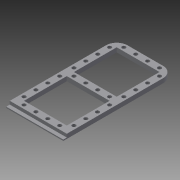
# Autodesk Inventor part: large edition 3 open
Saved by Autodesk Inventor 2015 (Build 190159000, 159)
## iProperties
Created: 2015-06-08
Part Number: large edition 3 open
Material: Generic
Document SubType Name: Modeling
Designer: Jason
Density: 1 g/cm^3
Appearance: Default
Author: Jason
Autodesk Inventor part; units mm, degrees
ref_plane "YZ Plane" through (0, 0, 0) normal (1, 0, 0) x (0, 1, 0)
ref_plane "XZ Plane" through (0, 0, 0) normal (0, 1, 0) x (-1, 0, 0)
ref_plane "XY Plane" through (0, 0, 0) normal (0, 0, 1) x (1, 0, 0)
sketch "Sketch1" plane through (0, 0, 0) normal (0, 0, 1) x (1, 0, 0)
  line L0 (0, 0) -> (90, 0)
  line L1 (90, 0) -> (90, -160)
  line L2 (90, -160) -> (0, -160)
  line L3 (0, -160) -> (0, 0)
  dimension "d0" = 90
  dimension "d1" = 160
  constraints: 8 end point, 2 parallel, 1 horizontal, 1 perpendicular
  measures "d0" distance of L1.end L2.end
  measures "d1" distance of L0.end L1.end
extrude "Extrusion1" add sketch "Sketch1" along normal blind 1.6
sketch "Sketch2" plane through (0, 0, 1.6) normal (0, 0, 1) x (1, 0, 0)
  line L0 (5, -5) -> (85, -5)
  line L1 (85, -5) -> (85, -15)
  line L2 (85, -15) -> (5, -15)
  line L3 (5, -15) -> (5, -5)
  line L4 (90, 0) -> (0, 0) projected
  line L5 (0, 0) -> (0, -160) projected
  line L6 (90, -160) -> (90, 0) projected
  line L7 (5, -5) -> (15, -5)
  line L8 (15, -5) -> (15, -155)
  line L9 (15, -155) -> (5, -155)
  line L10 (5, -155) -> (5, -5)
  line L11 (0, -160) -> (90, -160) projected
  line L12 (5, -155) -> (85, -155)
  line L13 (85, -155) -> (85, -145)
  line L14 (85, -145) -> (5, -145)
  line L15 (5, -145) -> (5, -155)
  line L16 (85, -5) -> (75, -5)
  line L17 (75, -5) -> (75, -155)
  line L18 (75, -155) -> (85, -155)
  line L19 (85, -155) -> (85, -5)
  line L20 (5, -75) -> (85, -75)
  line L21 (85, -75) -> (85, -85)
  line L22 (85, -85) -> (5, -85)
  line L23 (5, -85) -> (5, -75)
  dimension "d4" = 5
  dimension "d5" = 5
  dimension "d6" = 5
  dimension "d7" = 10
  dimension "d8" = 10
  dimension "d9" = 5
  dimension "d10" = 80
  dimension "d11" = 10
  dimension "d12" = 10
  dimension "d13" = 80
  dimension "d14" = 10
  dimension "d15" = 75
  constraints: 40 end point, 10 parallel, 5 horizontal, 5 perpendicular, 2 point on line
  measures "d4" distance between parallel lines of L4 L0
  measures "d5" distance between parallel lines of L5 L3
  measures "d6" distance between parallel lines of L6 L1
  measures "d7" distance between parallel lines of L2 L0
  measures "d8" distance of L8.end L9.end
  measures "d9" distance between parallel lines of L11 L9
  measures "d10" distance of L14.end L13.end
  measures "d11" distance of L13.end L12.end
  measures "d12" distance of L18.end L17.end
  measures "d13" distance of L21.end L22.end
  measures "d14" distance of L20.end L21.end
  measures "d15" distance between parallel lines of L20 L4
extrude "Extrusion2" add sketch "Sketch2" along normal blind 4.6 contours L0 L8 L2 L3 | L0 L17 L2 L8 | L2 L8 L20 L10 | L0 L1 L2 L17 | L20 L8 L22 L10 | L2 L19 L20 L17 | L20 L17 L22 L8 | L22 L8 L14 L10 | L20 L19 L22 L17 | L14 L8 L9 L10 | L22 L19 L14 L17 | L14 L17 L12 L8 | L14 L13 L12 L17
sketch "Sketch3" plane through (0, 0, 6.2) normal (0, 0, 1) x (1, 0, 0)
  circle A0 centre (20, -10) radius 2.6
  circle A1 centre (53.3333, -10) radius 2.6
  circle A2 centre (36.6667, -10) radius 2.6
  circle A3 centre (80, -140) radius 2.6
  circle A4 centre (80, -123.3333) radius 2.6
  circle A5 centre (80, -107) radius 2.6
  circle A6 centre (80, -90) radius 2.6
  circle A7 centre (70, -150) radius 2.6
  circle A8 centre (53.3333, -150) radius 2.6
  circle A9 centre (36.6667, -150) radius 2.6
  circle A10 centre (20, -150) radius 2.6
  circle A11 centre (10, -140) radius 2.6
  circle A12 centre (10, -123.3333) radius 2.6
  circle A13 centre (10, -106.6667) radius 2.6
  circle A14 centre (10, -90) radius 2.6
  circle A15 centre (70, -80) radius 2.6
  circle A16 centre (53.3333, -80) radius 2.6
  circle A17 centre (36.6667, -80) radius 2.6
  circle A18 centre (20, -80) radius 2.6
  circle A19 centre (80, -70) radius 2.6
  circle A20 centre (80, -53.3333) radius 2.6
  circle A21 centre (80, -36.6667) radius 2.6
  circle A22 centre (80, -20) radius 2.6
  circle A23 centre (10, -70) radius 2.6
  circle A24 centre (10, -53.3333) radius 2.6
  circle A25 centre (10, -36.6667) radius 2.6
  circle A26 centre (10, -20) radius 2.6
  circle A27 centre (70, -10) radius 2.6
  line L0 (85, -155) -> (5, -155) projected
  line L1 (85, -5) -> (5, -5) projected
  line L2 (5, -5) -> (5, -155) projected
  line L3 (15, -75) -> (15, -15) projected
  line L4 (75, -15) -> (75, -75) projected
  line L5 (15, -15) -> (75, -15) projected
  line L6 (85, -155) -> (85, -5) projected
  line L7 (15, -85) -> (75, -85) projected
  line L8 (15, -145) -> (15, -85) projected
  point P0 (0, 0)
  point P1 (90, -155)
  dimension "d18" = 5.2
  dimension "d20" = 5.2
  dimension "d21" = 5.2
  dimension "d22" = 5.2
  dimension "d23" = 5.2
  dimension "d24" = 5.2
  dimension "d25" = 5.2
  dimension "d26" = 5.2
  dimension "d27" = 5.2
  dimension "d28" = 5.2
  dimension "d29" = 5.2
  dimension "d30" = 5.2
  dimension "d31" = 5.2
  dimension "d32" = 5.2
  dimension "d33" = 5.2
  dimension "d34" = 5.2
  dimension "d35" = 5.2
  dimension "d36" = 5.2
  dimension "d37" = 5.2
  dimension "d38" = 5.2
  dimension "d39" = 5.2
  dimension "d40" = 5.2
  dimension "d41" = 5.2
  dimension "d42" = 5.2
  dimension "d43" = 5.2
  dimension "d44" = 5.2
  dimension "d45" = 5.2
  dimension "d47" = 5.2
  dimension "d48" = 5
  dimension "d49" = 5
  dimension "d50" = 5
  dimension "d51" = 5
  dimension "d52" = 5
  dimension "d53" = 5
  dimension "d55" = 5
  dimension "d56" = 16.6667
  dimension "d57" = 16.6667
  dimension "d58" = 5
  dimension "d59" = 16.6667
  dimension "d60" = 16.6667
  dimension "d61" = 16.6667
  dimension "d62" = 5
  dimension "d63" = 5
  dimension "d64" = 5
  dimension "d65" = 16.6667
  dimension "d66" = 16.6667
  dimension "d67" = 16.6667
  dimension "d68" = 5
  dimension "d73" = 16.6667
  dimension "d74" = 16.6667
  dimension "d75" = 16.6667
  constraints: 28 centre point
  measures "d18" diameter of A0
  measures "d20" diameter of A1
  measures "d21" diameter of A2
  measures "d22" diameter of A3
  measures "d23" diameter of A4
  measures "d24" diameter of A5
  measures "d25" diameter of A6
  measures "d26" diameter of A7
  measures "d27" diameter of A8
  measures "d28" diameter of A9
  measures "d29" diameter of A10
  measures "d30" diameter of A11
  measures "d31" diameter of A12
  measures "d32" diameter of A13
  measures "d33" diameter of A14
  measures "d34" diameter of A15
  measures "d35" diameter of A16
  measures "d36" diameter of A17
  measures "d37" diameter of A18
  measures "d38" diameter of A19
  measures "d39" diameter of A20
  measures "d40" diameter of A21
  measures "d41" diameter of A22
  measures "d42" diameter of A23
  measures "d43" diameter of A24
  measures "d44" diameter of A25
  measures "d45" diameter of A26
  measures "d47" diameter of A27
  measures "d48" distance from line of L1 A0.centre
  measures "d49" distance from line of L1 A2.centre
  measures "d50" distance from line of L1 A1.centre
  measures "d51" distance from line of L1 A27.centre
  measures "d52" distance from line of L2 A26.centre
  measures "d53" distance from line of L3 A0.centre
  measures "d55" distance from line of L4 A27.centre
  measures "d56" distance of A2.centre A0.centre
  measures "d57" distance of A1.centre A2.centre
  measures "d58" distance from line of L5 A26.centre
  measures "d59" distance of A26.centre A25.centre
  measures "d60" distance of A25.centre A24.centre
  measures "d61" distance of A24.centre A23.centre
  measures "d62" distance from line of A18.centre L3
  measures "d63" distance from line of L6 A22.centre
  measures "d64" distance from line of L7 A14.centre
  measures "d65" distance of A13.centre A14.centre
  measures "d66" distance of A12.centre A13.centre
  measures "d67" distance of A11.centre A12.centre
  measures "d68" distance from line of A10.centre L8
  measures "d73" distance of A17.centre A18.centre
  measures "d74" distance of A9.centre A10.centre
  measures "d75" distance of A8.centre A9.centre
extrude "Extrusion3" cut sketch "Sketch3" against normal through all contours A0 | A1 | A2 | A3 | A4 | A5 | A6 | A7 | A8 | A9 | A10 | A11 | A12 | A13 | A14 | A15 | A16 | A17 | A18 | A19 | A20 | A21 | A22 | A23 | A24 | A25 | A26 | A27
sketch "Sketch4" plane through (0, 0, 1.6) normal (0, 0, 1) x (1, 0, 0)
  line L0 (75, -15) -> (15, -15)
  line L1 (15, -15) -> (15, -75)
  line L2 (15, -75) -> (75, -75)
  line L3 (75, -75) -> (75, -15)
  line L4 (75, -85) -> (15, -85)
  line L5 (15, -85) -> (15, -145)
  line L6 (15, -145) -> (75, -145)
  line L7 (75, -145) -> (75, -85)
  line L8 (0, 0) -> (5, 0)
  line L9 (5, 0) -> (5, -155)
  line L10 (5, -155) -> (0, -155)
  line L11 (0, -155) -> (0, 0)
  line L12 (5, 0) -> (85, 0)
  line L13 (85, 0) -> (85, -5)
  line L14 (85, -5) -> (5, -5)
  line L15 (5, -5) -> (5, 0)
  line L16 (90, 0) -> (85, 0)
  line L17 (85, 0) -> (85, -155)
  line L18 (85, -155) -> (90, -155)
  line L19 (90, -155) -> (90, 0)
  line L20 (90, -160) -> (0, -160) projected
  line L21 (0, -155) -> (5, -155)
  line L22 (5, -155) -> (5, -160)
  line L23 (5, -160) -> (0, -160)
  line L24 (0, -160) -> (0, -155)
  line L25 (85, -155) -> (90, -155)
  line L26 (90, -155) -> (90, -160)
  line L27 (90, -160) -> (85, -160)
  line L28 (85, -160) -> (85, -155)
  constraints: 56 end point, 14 parallel, 7 horizontal, 7 perpendicular, 1 point on line
extrude "Extrusion4" cut sketch "Sketch4" against normal through all contours L3 L2 L1 L0 | L7 L6 L5 L4 | L8 L9 L10 L11 | L12 L13 L14 L9 | L10 L22 L20 L24 | L16 L19 L18 L17 L13 | L18 L26 L20 L28
fillet "Fillet1" radius 15 2 edges at (5, -5, 3.1) (85, -5, 3.1)
body "Solid1"
